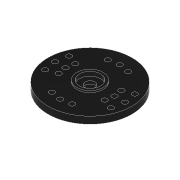
# Autodesk Inventor part: servo motor HS-7955TG round horn
Saved by Autodesk Inventor 2022 (Build 260153000, 153)
## iProperties
Created: 2017-12-19
Part Number: servo motor HS-7955TG round horn
Material: Generic
Document SubType Name: Modeling
Designer: s41607
Density: 1 g/cm^3
Appearance: Smooth - Black
Author: s41607
Autodesk Inventor part; units mm, degrees
ref_plane "YZ Plane" through (0, 0, 0) normal (1, 0, 0) x (0, 1, 0)
ref_plane "XZ Plane" through (0, 0, 0) normal (0, 1, 0) x (-1, 0, 0)
ref_plane "XY Plane" through (0, 0, 0) normal (0, 0, 1) x (1, 0, 0)
sketch "Sketch1" plane through (0, 0, 0) normal (0, 0, 1) x (1, 0, 0)
  line L0 (-16.8, 0) -> (16.8, 0) projected
  line L1 (0, 16.8) -> (0, -16.8) projected
  circle A0 centre (0, 0) radius 12
  dimension "d0" = 24
  constraints: 1 centre point, 1 coincident
  measures "d0" diameter of A0
extrude "Extrusion1" add sketch "Sketch1" along normal blind 2
sketch "Sketch2" plane through (0, 0, 0) normal (0, 0, 1) x (1, 0, 0)
  line L0 (0, 16.8) -> (0, -16.8) projected
  line L1 (-16.8, 0) -> (16.8, 0) projected
  circle A0 centre (0, 0) radius 4.5
  dimension "d3" = 9
  constraints: 1 centre point, 1 coincident
  measures "d3" diameter of A0
extrude "Extrusion2" add sketch "Sketch2" against normal blind 2.5
sketch "Sketch3" plane through (0, 0, -2.5) normal (0, 0, -1) x (-1, 0, 0)
  line L0 (-16.8, 0) -> (16.8, 0) projected
  line L1 (0, -16.8) -> (0, 16.8) projected
  circle A0 centre (0, 0) radius 2.9
  dimension "d6" = 5.8
  constraints: 1 centre point, 1 coincident
  measures "d6" diameter of A0
extrude "Extrusion3" cut sketch "Sketch3" against normal blind 3
sketch "Sketch4" plane through (0, 0, 2) normal (0, 0, 1) x (1, 0, 0)
  line L0 (0, 16.8) -> (0, -16.8) projected
  line L1 (-16.8, 0) -> (16.8, 0) projected
  circle A0 centre (0, 0) radius 3.75
  dimension "d9" = 7.5
  constraints: 1 centre point, 1 coincident
  measures "d9" diameter of A0
extrude "Extrusion4" add sketch "Sketch4" along normal blind 0.5
sketch "Sketch5" plane through (0, 0, 2.5) normal (0, 0, 1) x (1, 0, 0)
  line L0 (0, 16.8) -> (0, -16.8) projected
  line L1 (-16.8, 0) -> (16.8, 0) projected
  circle A0 centre (0, 0) radius 3
  dimension "d12" = 6
  constraints: 1 centre point, 1 coincident
  measures "d12" diameter of A0
extrude "Extrusion5" cut sketch "Sketch5" against normal blind 1.2
sketch "Sketch6" plane through (0, 0, 0) normal (0, 0, 1) x (1, 0, 0)
  line L0 (0, 16.8) -> (0, -16.8) projected
  line L1 (-16.8, 0) -> (16.8, 0) projected
  circle A0 centre (0, 0) radius 1.4
  dimension "d15" = 2.8
  constraints: 1 centre point, 1 coincident
  measures "d15" diameter of A0
extrude "Extrusion6" cut sketch "Sketch6" along normal through all
sketch "Sketch7" plane through (0, 0, 0) normal (0, 0, 1) x (1, 0, 0)
  line L0 (0, 16.8) -> (0, -16.8) projected
  line L1 (-16.8, 0) -> (16.8, 0) projected
  circle A0 centre (0, 0) radius 8.5 construction
  line L2 (-2.9072, 7.9874) -> (2.9072, -7.9874) construction
  line L3 (2.9072, 7.9874) -> (-2.9072, -7.9874) construction
  point P0 (0, 8.5)
  point P1 (0, -8.5)
  dimension "d18" = 17
  dimension "d20" = 20
  constraints: 6 point on circle, 4 end point, 3 symmetric about line, 2 point on line, 1 centre point, 1 coincident
  measures "d18" diameter of A0
  measures "d20" angle of L2 L0
hole "Hole1" at (0, 8.5, 0) at (0, -8.5, 0) at (2.9072, 7.9874, 0) at (-2.9072, 7.9874, 0) at (2.9072, -7.9874, 0) at (-2.9072, -7.9874, 0) direction (0, 0, 1) diameter 1.5 depth 8 tip angle 118
sketch "Sketch8" plane through (0, 0, 0) normal (0, 0, 1) x (1, 0, 0)
  line L0 (0, 16.8) -> (0, -16.8) projected
  line L1 (-16.8, 0) -> (16.8, 0) projected
  circle A0 centre (0, 0) radius 10 construction
  line L2 (9.3969, 3.4202) -> (-9.3969, -3.4202) construction
  line L3 (-9.3969, 3.4202) -> (9.3969, -3.4202) construction
  circle A1 centre (0, 0) radius 7 construction
  point P0 (-10, 0)
  point P1 (10, 0)
  point P2 (-6.5778, 2.3941)
  point P3 (-7, 0)
  point P4 (-6.5778, -2.3941)
  point P5 (6.5778, 2.3941)
  point P6 (7, 0)
  point P7 (6.5778, -2.3941)
  dimension "d28" = 20
  dimension "d30" = 40
  dimension "d31" = 14
  constraints: 12 point on circle, 8 point on line, 4 end point, 3 symmetric about line, 2 centre point, 2 coincident
  measures "d28" diameter of A0
  measures "d30" angle of L2 L3
  measures "d31" diameter of A1
hole "Hole2" at (-10, 0, 0) at (-9.3969, 3.4202, 0) at (-9.3969, -3.4202, 0) at (10, 0, 0) at (9.3969, 3.4202, 0) at (9.3969, -3.4202, 0) at (-6.5778, 2.3941, 0) at (-7, 0, 0) at (-6.5778, -2.3941, 0) at (6.5778, 2.3941, 0) at (7, 0, 0) at (6.5778, -2.3941, 0) direction (0, 0, 1) diameter 1.5 depth 8 tip angle 118
body "Solid1"
